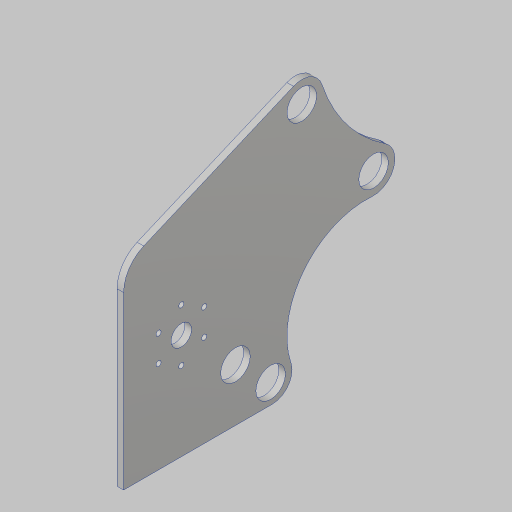
# Autodesk Inventor part: GI - 001
Saved by Autodesk Inventor 2023.5 (Build 275446000, 446)
## iProperties
Created: 2025-01-17
Part Number: GI - 001
Material: Aluminum 6061
Document SubType Name: Modeling
Designer: mavericks
Density: 2.7 g/cm^3
Appearance: Aluminum - Flat
Author: mavericks
Autodesk Inventor part; units mm, degrees
ref_plane "YZ Plane" through (0, 0, 0) normal (1, 0, 0) x (0, 1, 0)
ref_plane "XZ Plane" through (0, 0, 0) normal (0, 1, 0) x (-1, 0, 0)
ref_plane "XY Plane" through (0, 0, 0) normal (0, 0, 1) x (1, 0, 0)
sketch "Sketch2" plane through (0, 0, 0) normal (1, 0, 0) x (0, 1, 0)
  line L0 (63.5, 38.1) -> (-63.5, 38.1) construction
  line L1 (-63.5, 38.1) -> (-63.5, -38.1) construction
  line L2 (-63.5, -38.1) -> (63.5, -38.1) construction
  line L3 (63.5, -38.1) -> (63.5, 38.1) construction
  line L4 (63.5, 38.1) -> (-63.5, -38.1) construction
  line L5 (-63.5, 38.1) -> (63.5, -38.1) construction
  line L6 (-63.5, 38.1) -> (-76.2, 38.1) construction
  line L7 (-76.2, 38.1) -> (-76.2, -266.7) construction
  line L8 (-76.2, -266.7) -> (-63.5, -266.7) construction
  line L9 (-63.5, -266.7) -> (-63.5, 38.1) construction
  circle A0 centre (139.7, -401.3586) radius 57.15 construction
  circle A1 centre (-50.8, -103.823) radius 15.875 construction
  circle A2 centre (-19.05, -69.85) radius 25.4 construction
  circle A3 centre (76.2, -203.2) radius 63.5 construction
  circle A4 centre (76.2, -203.2) radius 14.2875
  circle A5 centre (166.7179, -133.8994) radius 38.1 construction
  circle A6 centre (166.7179, -133.8994) radius 14.2875
  circle A7 centre (-50.8, -103.823) radius 14.2875
  circle A8 centre (-19.05, -69.85) radius 14.2875
  line L10 (-69.85, 38.1) -> (-69.85, -105.4105)
  arc A9 (-50.8, -124.4605) -> (-44.3107, -123.4137) centre (-50.8, -103.823) ccw
  arc A10 (55.6237, -201.612) -> (93.4432, -214.5393) centre (76.2, -203.2) ccw
  arc A11 (173.1654, -153.5039) -> (185.7213, -125.8509) centre (166.7179, -133.8994) ccw
  arc A12 (55.6237, -201.612) -> (-44.3107, -123.4137) centre (-20.3504, -195.7487) ccw
  line L11 (-69.85, 38.1) -> (95.25, 38.1)
  line L12 (124.486, 18.7323) -> (185.7213, -125.8509)
  arc A13 (173.1654, -153.5039) -> (93.4432, -214.5393) centre (220.7773, -298.2757) ccw
  arc A14 (124.486, 18.7323) -> (95.25, 38.1) centre (95.25, 6.35) ccw
  arc A15 (-69.85, -105.4105) -> (-50.8, -124.4605) centre (-50.8, -105.4105) ccw
  line L13 (-57.15, 38.1) -> (-6.35, 38.1) construction
  line L14 (-6.35, 38.1) -> (-6.35, 444.5) construction
  line L15 (-6.35, 444.5) -> (-57.15, 444.5) construction
  line L16 (-57.15, 444.5) -> (-57.15, 38.1) construction
  point P0 (0, 0)
  point P1 (-14.3002, 165.1)
  point P2 (-49.1998, 165.1)
  point P3 (-14.3002, 190.5)
  point P4 (-49.1998, 190.5)
  point P5 (-14.3002, 215.9)
  point P6 (-49.1998, 215.9)
  point P7 (-14.3002, 241.3)
  point P8 (-49.1998, 241.3)
  dimension "d2" = 127
  dimension "d3" = 76.2
  dimension "d4" = 12.7
  dimension "d5" = 304.8
  dimension "d6" = 114.3
  dimension "d7" = 31.75
  dimension "d8" = 50.8
  dimension "d9" = 127
  dimension "d10" = 152.4
  dimension "d11" = 28.575
  dimension "d12" = 31.75
  dimension "d13" = 25.4
  dimension "d14" = 46.4998
  dimension "d15" = 44.45
  dimension "d16" = 165.1
  dimension "d17" = 76.2
  dimension "d18" = 114.0003
  dimension "d20" = 28.575
  dimension "d21" = 28.575
  dimension "d22" = 28.575
  dimension "d23" = 6.35
  dimension "d24" = 6.35
  dimension "d25" = 6.35
  dimension "d26" = 76.2
  dimension "d28" = 165.1
  dimension "d29" = 152.4
  dimension "d30" = 31.75
  dimension "d35" = 19.05
  dimension "d40" = 50.8
  dimension "d41" = 19.05
  dimension "d42" = 406.4
  dimension "d43" = 127
  dimension "d44" = 7.9502
  dimension "d45" = 7.9502
  dimension "d48" = 25.4
  dimension "d70" = 196.4995
  constraints: 34 end point, 16 centre point, 14 point on circle, 10 tangent, 6 parallel, 4 coincident, 4 perpendicular, 3 horizontal, 3 midpoint, 1 horizontal alignment, 1 point on line, 1 vertical, 6 other
  measures "d2" distance of L2.end L1.end
  measures "d3" distance of L1.end L0.end
  measures "d4" distance of L8.end L7.end
  measures "d5" distance of L7.end L6.end
  measures "d6" diameter of A0
  measures "d7" diameter of A1
  measures "d8" diameter of A2
  measures "d9" diameter of A3
  measures "d10" distance from line of A3.centre L7
  measures "d11" diameter of A4
  measures "d12" distance from line of A2.centre L2
  measures "d13" distance from line of L7 A1.centre
  measures "d14" distance of A2.centre A1.centre
  measures "d15" distance from line of L9 A2.centre
  measures "d16" distance from line of L2 A3.centre
  measures "d17" diameter of A5
  measures "d18" distance of A3.centre A5.centre
  measures "d20" diameter of A6
  measures "d21" diameter of A7
  measures "d22" diameter of A8
  measures "d23" radial gap between concentric circles of A7 A9
  measures "d24" radial gap between concentric circles of A4 A10
  measures "d25" radial gap between concentric circles of A6 A11
  measures "d26" radius of A12
  measures "d28" distance of L11.end L10.start
  measures "d29" radius of A13
  measures "d30" radius of A14
  measures "d35" radius of A15
  measures "d40" distance of L15.end L14.end
  measures "d41" distance between parallel lines of L16 L7
  measures "d42" distance of L15.end L13.start
  measures "d43" distance from line of L0 point (-14.3, 165.1)
  measures "d44" distance from line of L14 point (-14.3, 165.1)
  measures "d45" distance from line of L16 point (-49.2, 165.1)
  measures "d48" distance of point (-14.3, 165.1) point (-14.3, 190.5)
  measures "d70" distance of A2.centre A5.centre
extrude "Extrusion1" add sketch "Sketch2" along normal blind 6.35
sketch "Sketch3" plane through (6.35, 0, 0) normal (1, 0, 0) x (0, 0, -1)
  line L0 (-38.1, 63.5) -> (38.1, 63.5) construction
  line L1 (38.1, 63.5) -> (38.1, -63.5) construction
  line L2 (38.1, -63.5) -> (-38.1, -63.5) construction
  line L3 (-38.1, -63.5) -> (-38.1, 63.5) construction
  line L4 (-38.1, 63.5) -> (38.1, -63.5) construction
  line L5 (38.1, 63.5) -> (-38.1, -63.5) construction
  line L6 (-38.1, -69.85) -> (105.4105, -69.85) construction
  line L7 (-38.1, 95.25) -> (-38.1, -69.85) construction
  point P0 (0, 0)
  point P1 (0, 0)
  dimension "d36" = 76.2
  dimension "d37" = 127
  dimension "d38" = 6.35
  dimension "d39" = 0
  constraints: 12 end point, 2 midpoint, 2 parallel, 1 horizontal, 1 perpendicular
  measures "d36" distance of L1.end L2.end
  measures "d37" distance of L0.end L1.end
  measures "d38" distance between parallel lines of L6 L2
  measures "d39" distance between parallel lines of L7 L3
sketch "Sketch4" plane through (0, 0, 0) normal (-1, 0, 0) x (0, 0, 1)
  circle A0 centre (-17.5992, 31.75) radius 9.906
  circle A1 centre (-203.2, 76.2) radius 14.2875 projected
  circle A2 centre (-133.8994, 166.7179) radius 14.2875 projected
  circle A3 centre (-103.823, -50.8) radius 14.2875 projected
  circle A4 centre (-69.85, -19.05) radius 14.2875 projected
  arc A5 (38.1, 95.25) -> (18.7323, 124.486) centre (6.35, 95.25) ccw projected
  line L0 (38.1, 95.25) -> (38.1, -69.85) projected
  line L1 (38.1, -69.85) -> (-105.4105, -69.85) projected
  arc A6 (-124.4605, -50.8) -> (-105.4105, -69.85) centre (-105.4105, -50.8) ccw projected
  arc A7 (-123.4137, -44.3107) -> (-124.4605, -50.8) centre (-103.823, -50.8) ccw projected
  arc A8 (-123.4137, -44.3107) -> (-201.612, 55.6237) centre (-195.7487, -20.3504) ccw projected
  arc A9 (-214.5393, 93.4432) -> (-201.612, 55.6237) centre (-203.2, 76.2) ccw projected
  arc A10 (-214.5393, 93.4432) -> (-153.5039, 173.1654) centre (-298.2757, 220.7773) ccw projected
  arc A11 (-125.8509, 185.7213) -> (-153.5039, 173.1654) centre (-133.8994, 166.7179) ccw projected
  line L2 (-125.8509, 185.7213) -> (18.7323, 124.486) projected
  circle A12 centre (-203.2, 76.2) radius 14.2875 projected
  circle A13 centre (-133.8994, 166.7179) radius 14.2875 projected
  circle A14 centre (-103.823, -50.8) radius 14.2875 projected
  circle A15 centre (-69.85, -19.05) radius 14.2875 projected
  line L3 (38.1, 95.25) -> (38.1, -69.85) projected
  line L4 (38.1, -69.85) -> (-105.4105, -69.85) projected
  circle A16 centre (-17.5992, 31.75) radius 25.4 construction
  arc A17 (38.1, 95.25) -> (18.7323, 124.486) centre (6.35, 95.25) ccw projected
  arc A18 (-124.4605, -50.8) -> (-105.4105, -69.85) centre (-105.4105, -50.8) ccw projected
  arc A19 (-123.4137, -44.3107) -> (-124.4605, -50.8) centre (-103.823, -50.8) ccw projected
  arc A20 (-123.4137, -44.3107) -> (-201.612, 55.6237) centre (-195.7487, -20.3504) ccw projected
  arc A21 (-214.5393, 93.4432) -> (-201.612, 55.6237) centre (-203.2, 76.2) ccw projected
  arc A22 (-214.5393, 93.4432) -> (-153.5039, 173.1654) centre (-298.2757, 220.7773) ccw projected
  arc A23 (-125.8509, 185.7213) -> (-153.5039, 173.1654) centre (-133.8994, 166.7179) ccw projected
  line L5 (-125.8509, 185.7213) -> (18.7323, 124.486) projected
  point P0 (0, 0)
  point P1 (-17.5992, 57.15)
  point P2 (-39.5962, 44.45)
  point P3 (-39.5962, 19.05)
  point P4 (-17.5992, 6.35)
  point P5 (4.3978, 19.05)
  point P6 (4.3978, 44.45)
  dimension "d58" = 50.8
  dimension "d53" = 19.812
  dimension "d54" = 72.8751
  dimension "d55" = 101.6
  dimension "d61" = 360
  constraints: 2 vertical alignment, 1 centre point, 1 coincident, 9 other
  measures "d53" diameter of A0
  measures "d54" distance of A0.centre A4.centre
  measures "d55" distance from line of L1 A0.centre
extrude "Extrusion2" cut sketch "Sketch4" against normal blind 25.4 contours A0
hole "Hole1" at (0, 57.15, -17.5992) at (0, 44.45, -39.5962) at (0, 19.05, -39.5962) at (0, 6.35, -17.5992) at (0, 19.05, 4.3978) at (0, 44.45, 4.3978) direction (1, 0, 0) diameter 5.1054 end through all clearance for "Flat Head Machine Screw (82)" size "#10" standard "Ansi Unified Screw Threads"
body "Solid1"
